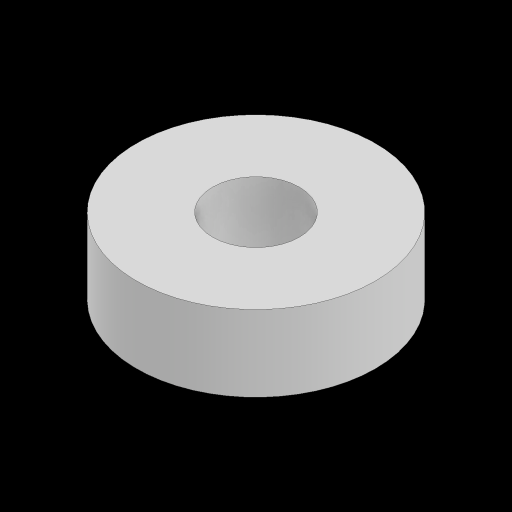
# Autodesk Inventor part: 608bearing
Saved by Autodesk Inventor 2023 (Build 270158030, 158C)
## iProperties
Created: 2022-08-15
Part Number: 608bearing
Material: Generic
Document SubType Name: Modeling
Designer: kumpu
Density: 1 g/cm^3
Appearance: Default
Author: kumpu
Autodesk Inventor part; units mm, degrees
ref_plane "YZ Plane" through (0, 0, 0) normal (1, 0, 0) x (0, 1, 0)
ref_plane "XZ Plane" through (0, 0, 0) normal (0, 1, 0) x (-1, 0, 0)
ref_plane "XY Plane" through (0, 0, 0) normal (0, 0, 1) x (1, 0, 0)
sketch "Sketch1" plane through (0, 0, 0) normal (0, 0, 1) x (1, 0, 0)
  line L0 (4, 3.5) -> (11, 3.5)
  line L1 (11, 3.5) -> (11, -3.5)
  line L2 (11, -3.5) -> (4, -3.5)
  line L3 (4, -3.5) -> (4, 3.5)
  line L4 (4, 3.5) -> (11, -3.5) construction
  line L5 (11, 3.5) -> (4, -3.5) construction
  line L6 (4, 0) -> (0, 0) construction
  line L7 (0, 0) -> (0, 3.5) construction
  point P0 (7.5, 0)
  dimension "d0" = 7
  dimension "d1" = 7
  dimension "d2" = 4
  constraints: 16 end point, 3 midpoint, 2 parallel, 2 perpendicular, 1 horizontal, 1 point on line, 1 vertical
  measures "d0" distance of L1.end L2.end
  measures "d1" distance of L0.end L1.end
  measures "d2" distance of L6.start L6.end
revolve "Revolution1" add sketch "Sketch1" angle 360 about axis through (0, 0, 0) along (0, 1, 0)
body "Solid1"
